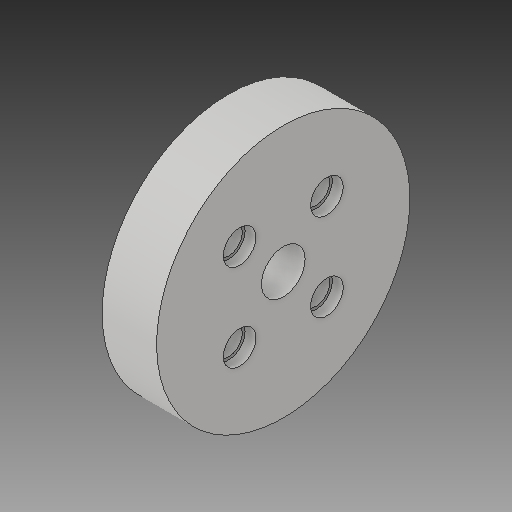
# Autodesk Inventor part: Tapon 1
Saved by Autodesk Inventor 2018.3 (Build 223284000, 284)
## iProperties
Created: 2019-03-12
Part Number: Tapon 1
Material: Generic
Document SubType Name: Modeling
Designer: Mario
Density: 1 g/cm^3
Appearance: Default
Author: Mario
Autodesk Inventor part; units mm, degrees
ref_plane "YZ Plane" through (0, 0, 0) normal (1, 0, 0) x (0, 1, 0)
ref_plane "XZ Plane" through (0, 0, 0) normal (0, 1, 0) x (-1, 0, 0)
ref_plane "XY Plane" through (0, 0, 0) normal (0, 0, 1) x (1, 0, 0)
sketch "Sketch1" plane through (0, 0, 0) normal (1, 0, 0) x (0, 1, 0)
  circle A0 centre (0, 0) radius 23.2155
  circle A1 centre (0, 0) radius 23.2155 projected
  dimension "d0" = 46.431
  dimension "d21" = 46.431
  constraints: 1 centre point, 1 coincident
  measures "d0" diameter of A0
  measures "d21" diameter of A1
extrude "Extrusion1" add sketch "Sketch1" along normal blind 10
sketch "Sketch2" plane through (10, 0, 0) normal (1, 0, 0) x (0, 0, -1)
  point P0 (0, 0)
  point P1 (-8, 8)
  point P2 (8, 8)
  point P3 (8, -8)
  point P4 (-8, -8)
  dimension "d3" = 8
  dimension "d4" = 8
  dimension "d5" = 16
  dimension "d6" = 16
  constraints: 2 horizontal alignment, 2 vertical alignment
  measures "d3" horizontal distance of point (0, 0) point (-8, 8)
  measures "d4" horizontal distance of point (0, 0) point (-8, 8)
  measures "d5" distance of point (-8, -8) point (-8, 8)
  measures "d6" distance of point (8, -8) point (-8, -8)
hole "Hole1" at (10, 8, 8) at (10, 8, -8) at (10, -8, -8) at (10, -8, 8) direction (-1, 0, 0) diameter 5 end through all counterbore diameter 6 counterbore depth 2
sketch "Sketch3" plane through (10, 0, 0) normal (1, 0, 0) x (0, 0, -1)
  point P0 (0, 0)
  point P1 (0, 0)
  constraints: 1 coincident
hole "Hole2" at (10, 0, 0) direction (-1, 0, 0) diameter 8 end through all
equation "\"d0\" = d21"
equation "\"d5\" = 2 * d3"
equation "\"d6\" = d5"
body "Solid1"
